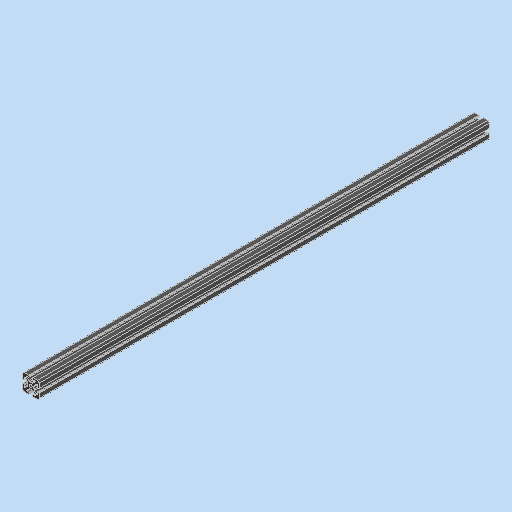
# Autodesk Inventor part: T-SLOT 4040 B-Type 1087mm
Saved by Autodesk Inventor 2023.2 (Build 272271000, 271)
## iProperties
Created: 2023-11-21
Part Number: T-SLOT 4040 B-Type 1087mm
Material: Generisch
Document SubType Name: Modeling
Designer: Nils Bade
Density: 1 g/cm^3
Appearance: Vorgabe(1)
Auf Bestellliste: False
Listed: True
Author: Nils Bade
Autodesk Inventor part; units mm, degrees
ref_plane "YZ Plane" through (0, 0, 0) normal (1, 0, 0) x (0, 1, 0)
ref_plane "XZ Plane" through (0, 0, 0) normal (0, 1, 0) x (-1, 0, 0)
ref_plane "XY Plane" through (0, 0, 0) normal (0, 0, 1) x (1, 0, 0)
sketch "T-Slot 4040 Base" plane through (0, 0, 0) normal (0, 0, 1) x (1, 0, 0)
  line L0 (-28, 0) -> (28, 0) construction
  line L1 (0, -28) -> (0, 28) construction
  circle A0 centre (0, 0) radius 3.4
  line L2 (-7.5, -7.5) -> (7.5, -7.5)
  line L3 (7.5, -7.5) -> (7.5, 7.5)
  line L4 (7.5, 7.5) -> (-7.5, 7.5)
  line L5 (-7.5, 7.5) -> (-7.5, -7.5)
  line L6 (-7.5, -7.5) -> (7.5, 7.5) construction
  line L7 (7.5, -7.5) -> (-7.5, 7.5) construction
  line L8 (20, 4) -> (15.5, 4)
  line L9 (15.5, 4) -> (15.5, 12)
  line L10 (15.5, 12) -> (7.5, 4)
  line L11 (4, 20) -> (4, 15.5)
  line L12 (4, 15.5) -> (12, 15.5)
  line L13 (12, 15.5) -> (4, 7.5)
  line L14 (7.5, -7.5) -> (-7.5, -7.5)
  arc A1 (15.5, 9.5858) -> (13.7929, 10.2929) centre (14.5, 9.5858) ccw
  arc A2 (10.2929, 13.7929) -> (9.5858, 15.5) centre (9.5858, 14.5) ccw
  line L15 (-20, 20) -> (20, 20)
  line L16 (20, 20) -> (20, -20)
  line L17 (20, -20) -> (-20, -20)
  line L18 (-20, -20) -> (-20, 20)
  line L19 (-20, 20) -> (20, -20) construction
  line L20 (20, 20) -> (-20, -20) construction
  line L21 (-4, 15.5) -> (-12, 15.5)
  arc A3 (-9.5858, 15.5) -> (-10.2929, 13.7929) centre (-9.5858, 14.5) ccw
  line L22 (-12, 15.5) -> (-4, 7.5)
  line L23 (-15.5, 12) -> (-7.5, 4)
  line L24 (-20, 4) -> (-15.5, 4)
  arc A4 (-13.7929, 10.2929) -> (-15.5, 9.5858) centre (-14.5, 9.5858) ccw
  line L25 (-15.5, 4) -> (-15.5, 12)
  line L26 (-4, 20) -> (-4, 15.5)
  line L27 (-15.5, -4) -> (-15.5, -12)
  arc A5 (-15.5, -9.5858) -> (-13.7929, -10.2929) centre (-14.5, -9.5858) ccw
  line L28 (-15.5, -12) -> (-7.5, -4)
  line L29 (-12, -15.5) -> (-4, -7.5)
  line L30 (-4, -20) -> (-4, -15.5)
  arc A6 (-10.2929, -13.7929) -> (-9.5858, -15.5) centre (-9.5858, -14.5) ccw
  line L31 (-4, -15.5) -> (-12, -15.5)
  line L32 (-20, -4) -> (-15.5, -4)
  line L33 (4, -15.5) -> (12, -15.5)
  arc A7 (9.5858, -15.5) -> (10.2929, -13.7929) centre (9.5858, -14.5) ccw
  line L34 (12, -15.5) -> (4, -7.5)
  line L35 (15.5, -12) -> (7.5, -4)
  line L36 (20, -4) -> (15.5, -4)
  arc A8 (13.7929, -10.2929) -> (15.5, -9.5858) centre (14.5, -9.5858) ccw
  line L37 (15.5, -4) -> (15.5, -12)
  line L38 (4, -20) -> (4, -15.5)
  point P0 (4.9274, 7.75)
  point P1 (9.5858, 15.5)
  point P2 (-20, 20)
  point P3 (-7.5, -7.5)
  point P4 (-20, -20)
  point P5 (7.5, -7.5)
  point P6 (20, -20)
  point P7 (-9.5858, -15.5)
  point P8 (-4, -7.5)
  point P9 (15.5, -9.5858)
  point P10 (7.5, -4)
  point P11 (-15.5, 9.5858)
  point P12 (-4, 7.5)
  dimension "d35" = 6.8
  dimension "d37" = 12
  dimension "d38" = 1
  dimension "d43" = 40
  dimension "d44" = 40
  dimension "d45" = 4.5
  dimension "d46" = 4
  dimension "d53" = 360
  constraints: 74 end point, 16 point on circle, 15 point on line, 9 centre point, 6 midpoint, 5 parallel, 5 perpendicular, 3 horizontal, 3 symmetric about line, 2 tangent, 101 other
  measures "d35" diameter of A0
  measures "d37" distance from line of L0 L9.end
  measures "d38" radius of A1
  measures "d43" distance of L16.end L17.end
  measures "d44" distance of L15.end L16.end
  measures "d45" distance between parallel lines of L16 L9
  measures "d46" distance between parallel lines of L0 L8
extrude "Extrusion1" add sketch "T-Slot 4040 Base" along normal blind 1087 contours L5 L4 L3 L2 | L2 L29 L31 L30 L17 L18 L32 L27 L28 L5 | L2 L3 L35 L37 L36 L16 L17 L38 L33 L34 | A6 L31 L29 | L23 L25 L24 L18 L15 L26 L21 L22 L4 L5 | L28 L27 A5 | L34 L33 A7 | A4 L25 L23 | L3 L4 L13 L12 L11 L15 L16 L8 L9 L10 | A8 L37 L35 | L22 L21 A3 | L10 L9 A1 | A2 L12 L13
fillet "Rundung1" radius 1 16 edges at (4, 15.5, 543.5) (15.5, 4, 543.5) (20, 4, 543.5) (4, 20, 543.5) (-20, 4, 543.5) (-15.5, 4, 543.5) (-4, 15.5, 543.5) (-4, 20, 543.5) (-4, -15.5, 543.5) (-4, -20, 543.5) (4, -15.5, 543.5) (4, -20, 543.5) (15.5, -4, 543.5) (20, -4, 543.5) (-20, -4, 543.5) (-15.5, -4, 543.5)
fillet "Rundung2" radius 4 12 edges at (4, 7.5, 543.5) (7.5, 4, 543.5) (-20, 20, 543.5) (-20, -20, 543.5) (20, 20, 543.5) (20, -20, 543.5) (7.5, -4, 543.5) (-7.5, -4, 543.5) (-7.5, 4, 543.5) (4, -7.5, 543.5) (-4, -7.5, 543.5) (-4, 7.5, 543.5)
